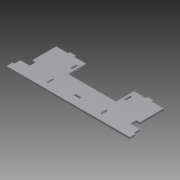
# Autodesk Inventor part: OpenROV 2_2a Forward Bulkhead
Saved by Autodesk Inventor 2011 (Build 150239000, 239)
## iProperties
Created: 2011-09-23
Part Number: OpenROV 2_2a Forward Bulkhead
Document SubType Name: Modeling
Designer: user
Density: 1 g/cm^3
Author: user
Autodesk Inventor part; units mm, degrees
ref_plane "YZ Plane" through (0, 0, 0) normal (1, 0, 0) x (0, 1, 0)
ref_plane "XZ Plane" through (0, 0, 0) normal (0, 1, 0) x (-1, 0, 0)
ref_plane "XY Plane" through (0, 0, 0) normal (0, 0, 1) x (1, 0, 0)
sketch "Sketch1" plane through (0, 0, 0) normal (0, 0, 1) x (1, 0, 0)
  line L0 (-40, 0) -> (-40, -29)
  line L1 (-39, -30) -> (39, -30)
  line L2 (40, -29) -> (40, 0)
  line L3 (100, -50) -> (100, -60)
  line L4 (100, -60) -> (103, -60)
  line L5 (103, -60) -> (103, -69)
  line L6 (102, -70) -> (-102, -70)
  line L7 (-103, -69) -> (-103, -60)
  line L8 (-103, -60) -> (-100, -60)
  line L9 (-100, -60) -> (-100, -50)
  line L10 (-60, 0) -> (-60, 3)
  line L11 (-60, 3) -> (-70, 3)
  line L12 (-70, 3) -> (-70, 0)
  line L13 (-90, 0) -> (-70, 0)
  line L14 (-60, 0) -> (-40, 0)
  line L15 (70, 0) -> (70, 3)
  line L16 (70, 3) -> (60, 3)
  line L17 (60, 3) -> (60, 0)
  line L18 (40, 0) -> (60, 0)
  line L19 (70, 0) -> (90, 0)
  arc A0 (-103, -69) -> (-102, -70) centre (-102, -69) ccw
  arc A1 (102, -70) -> (103, -69) centre (102, -69) ccw
  arc A2 (39, -30) -> (40, -29) centre (39, -29) ccw
  arc A3 (-40, -29) -> (-39, -30) centre (-39, -29) ccw
  line L20 (-90, -40) -> (-84, -40)
  line L21 (-84, -40) -> (-84, -50)
  line L22 (90, -40) -> (84, -40)
  line L23 (84, -40) -> (84, -50)
  line L24 (-43.5, -10) -> (-46.5, -10)
  line L25 (-46.5, -10) -> (-46.5, -20)
  line L26 (-46.5, -20) -> (-43.5, -20)
  line L27 (-43.5, -20) -> (-43.5, -10)
  line L28 (43.5, -10) -> (46.5, -10)
  line L29 (46.5, -10) -> (46.5, -20)
  line L30 (46.5, -20) -> (43.5, -20)
  line L31 (43.5, -20) -> (43.5, -10)
  line L32 (-46.5, -50) -> (-43.5, -50)
  line L33 (-43.5, -50) -> (-43.5, -60)
  line L34 (-43.5, -60) -> (-46.5, -60)
  line L35 (-46.5, -60) -> (-46.5, -50)
  line L36 (43.5, -50) -> (46.5, -50)
  line L37 (46.5, -50) -> (46.5, -60)
  line L38 (46.5, -60) -> (43.5, -60)
  line L39 (43.5, -60) -> (43.5, -50)
  line L40 (-5, -53) -> (5, -53)
  line L41 (5, -53) -> (5, -56)
  line L42 (5, -56) -> (-5, -56)
  line L43 (-5, -56) -> (-5, -53)
  line L44 (-90, 0) -> (-90, -40)
  line L45 (-84, -50) -> (-100, -50)
  line L46 (84, -50) -> (100, -50)
  line L47 (90, -40) -> (90, 0)
  point P0 (0, 0)
  point P1 (-40, -30)
  point P2 (40, -30)
  point P3 (103, -70)
  point P4 (-103, -70)
  dimension "d0" = 80
  dimension "d1" = 30
  dimension "d2" = 50
  dimension "d4" = 10
  dimension "d5" = 10
  dimension "d7" = 10
  dimension "d8" = 10
  dimension "d10" = 50
  dimension "d13" = 3
  dimension "d14" = 3
  dimension "d15" = 3
  dimension "d16" = 10
  dimension "d18" = 10
  dimension "d20" = 3
  dimension "d21" = 40
  dimension "d22" = 206
  dimension "d23" = 30
  dimension "d24" = 40
  dimension "d27" = 1
  dimension "d28" = 10
  dimension "d29" = 6
  dimension "d31" = 40
  dimension "d32" = 10
  dimension "d33" = 6
  dimension "d35" = 40
  dimension "d39" = 10
  dimension "d40" = 3
  dimension "d41" = 10
  dimension "d42" = 3
  dimension "d44" = 10
  dimension "d45" = 10
  dimension "d50" = 3
  dimension "d51" = 10
  dimension "d52" = 10
  dimension "d54" = 3
  dimension "d55" = 10
  dimension "d56" = 10
  dimension "d60" = 10
  dimension "d61" = 3
  dimension "d62" = 17
  dimension "d66" = 40
  dimension "d67" = 40
  dimension "d68" = 16
  dimension "d69" = 20
  dimension "d70" = 20
  dimension "d71" = 3.5
  dimension "d72" = 3.5
  dimension "d73" = 3.5
  dimension "d74" = 3.5
  constraints: 96 end point, 26 parallel, 11 perpendicular, 9 horizontal, 8 point on circle, 8 point on line, 8 tangent, 4 centre point, 4 collinear, 3 equal radius
  measures "d0" distance of point (-40, -30) point (40, -30)
  measures "d1" distance of point (40, -30) L2.end
  measures "d2" distance of L2.end L19.end
  measures "d4" distance of L3.start L3.end
  measures "d5" distance of L4.end point (103, -70)
  measures "d7" distance of point (-103, -70) L7.end
  measures "d8" distance of L8.end L9.end
  measures "d10" distance of L13.start L0.start
  measures "d13" distance of L3.end L4.end
  measures "d14" distance of L7.end L8.end
  measures "d15" distance between parallel lines of L11 L13
  measures "d16" distance of L10.end L11.end
  measures "d18" distance of L15.end L16.end
  measures "d20" distance between parallel lines of L19 L16
  measures "d21" distance between parallel lines of L6 L1
  measures "d22" distance of point (103, -70) point (-103, -70)
  measures "d23" distance from line of point (0, 0) L1
  measures "d24" distance from line of point (0, 0) L2
  measures "d27" radius of A0
  measures "d28" distance of L20.end L21.end
  measures "d29" distance of L20.start L20.end
  measures "d31" distance between parallel lines of L14 L20
  measures "d32" distance of L22.end L23.end
  measures "d33" distance of L22.start L22.end
  measures "d35" distance between parallel lines of L18 L22
  measures "d39" distance of L26.end L24.start
  measures "d40" distance of L25.end L26.end
  measures "d41" distance between parallel lines of L14 L24
  measures "d42" distance of L28.start L28.end
  measures "d44" distance of L28.end L29.end
  measures "d45" distance between parallel lines of L18 L28
  measures "d50" distance of L33.end L34.end
  measures "d51" distance of L34.end L32.start
  measures "d52" distance between parallel lines of L6 L34
  measures "d54" distance of L37.end L38.end
  measures "d55" distance of L36.end L37.end
  measures "d56" distance between parallel lines of L6 L38
  measures "d60" distance of L41.end L42.end
  measures "d61" distance of L40.end L41.end
  measures "d62" distance between parallel lines of L6 L40
  measures "d66" distance of L13.start L20.start
  measures "d67" distance of L22.start L19.end
  measures "d68" distance of L23.end L3.start
  measures "d69" distance between parallel lines of L44 L12
  measures "d70" distance between parallel lines of L47 L15
  measures "d71" distance between parallel lines of L2 L31
  measures "d72" distance between parallel lines of L0 L27
  measures "d73" distance between parallel lines of L0 L33
  measures "d74" distance between parallel lines of L39 L2
extrude "Extrusion6" add sketch "Sketch1" along normal blind 3
body "Solid6"
